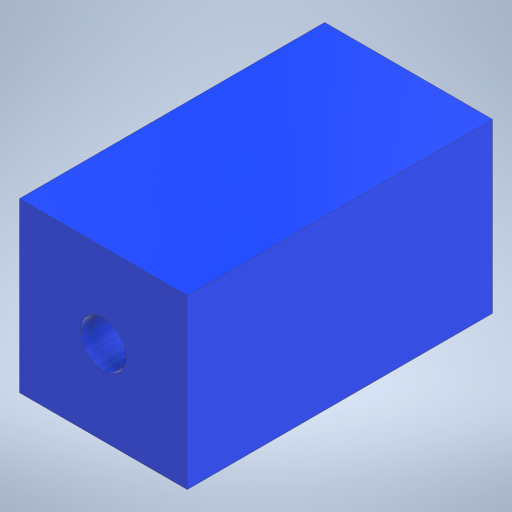
# Autodesk Inventor part: Aluminium-Connector_Lengan panjangk
Saved by Autodesk Inventor 2024 (Build 280153000, 153)
## iProperties
Created: 2023-09-10
Part Number: Aluminium-Connector_Lengan panjangk
Material: Generic
Document SubType Name: Modeling
Designer: AlfaNooraFithria
Density: 1 g/cm^3
Appearance: Default
Author: AlfaNooraFithria
Autodesk Inventor part; units mm, degrees
ref_plane "YZ Plane" through (0, 0, 0) normal (1, 0, 0) x (0, 1, 0)
ref_plane "XZ Plane" through (0, 0, 0) normal (0, 1, 0) x (-1, 0, 0)
ref_plane "XY Plane" through (0, 0, 0) normal (0, 0, 1) x (1, 0, 0)
sketch "Sketch1" plane through (0, 0, 0) normal (0, 0, 1) x (1, 0, 0)
  line L0 (0, 0) -> (11, 0)
  line L1 (11, 0) -> (11, 11)
  line L2 (11, 11) -> (0, 11)
  line L3 (0, 11) -> (0, 0)
  circle A0 centre (5.5, 5.5) radius 1.5
  dimension "d0" = 11
  dimension "d1" = 11
  dimension "d2" = 3
  constraints: 8 end point, 2 parallel, 1 centre point, 1 horizontal, 1 perpendicular
  measures "d0" distance of L2.end L1.end
  measures "d1" distance of L1.end L0.end
  measures "d2" diameter of A0
extrude "Extrusion1" add sketch "Sketch1" against normal blind 20
body "Solid1"
